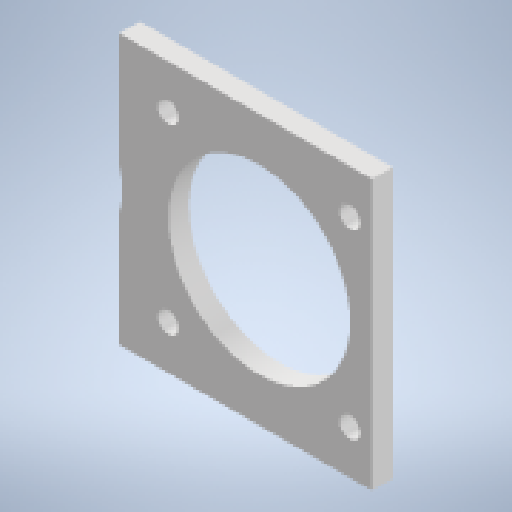
# Autodesk Inventor part: Shaft stabilizer
Saved by Autodesk Inventor 2024 (Build 280153000, 153)
## iProperties
Created: 2024-04-03
Part Number: Shaft stabilizer
Material: Generic
Document SubType Name: Modeling
Designer: drew
Density: 1 g/cm^3
Appearance: Default
Author: drew
Autodesk Inventor part; units mm, degrees
ref_plane "YZ Plane" through (0, 0, 0) normal (1, 0, 0) x (0, 1, 0)
ref_plane "XZ Plane" through (0, 0, 0) normal (0, 1, 0) x (-1, 0, 0)
ref_plane "XY Plane" through (0, 0, 0) normal (0, 0, 1) x (1, 0, 0)
sketch "Sketch1" plane through (0, 0, 0) normal (0, 0, 1) x (1, 0, 0)
  circle A0 centre (17.25, 15.5) radius 1.75 projected
  line L0 (-22.0887, 3.6324) -> (-22.0887, 23) projected
  arc A1 (-22.0887, -3.6324) -> (-22.0887, 3.6324) centre (-33, 0) ccw projected
  line L1 (-22.0887, -23) -> (-22.0887, -3.6324) projected
  line L2 (21, -23) -> (-22.0887, -23) projected
  line L3 (21, 23) -> (21, -23) projected
  line L4 (-22.0887, 23) -> (21, 23) projected
  circle A2 centre (17.25, -15.5) radius 1.75 projected
  circle A3 centre (-13.75, -15.5) radius 1.75 projected
  circle A4 centre (-13.75, 15.5) radius 1.75 projected
  circle A5 centre (17.25, 15.5) radius 1.75 projected
  circle A6 centre (1.75, 0) radius 15.5 projected
  point P0 (0, 0)
extrude "Extrusion1" add sketch "Sketch1" along normal blind 3.5
ref_plane "Work Plane1" through (-33, 0, -23) normal (0, 0, 1) x (1, 0, 0)
sketch "Sketch2" plane through (-33, 0, -23) normal (0, 0, 1) x (1, 0, 0)
  spline S0 degree 3 poles (-10, 18.589) (-10, 18.7259) (-9.9842, 18.8622) (-9.9495, 19.0178) (-9.9443, 19.0395) (-9.8997, 19.2118) (-9.8438, 19.3561) (-9.7735, 19.4974) (-9.7728, 19.4987) (-9.7722, 19.5) knots 0 0 0 0 0.433174 0.433174 0.503481 0.503481 0.995358 0.995358 1 1 1 1
  line L0 (-10, 12.8288) -> (-10, 18.589)
  arc A0 (-15, 7.8288) -> (-10, 12.8288) centre (-15, 12.8288) ccw
  line L1 (-15, 7.8288) -> (-28.448, 7.8288)
  arc A1 (-28.448, 7.8288) -> (-34.7485, 4.6469) centre (-28.448, 0) ccw
  line L2 (-34.7485, 4.6469) -> (-47.9719, -13.2822)
  arc A2 (-47.9719, -13.2822) -> (-48.948, -16.25) centre (-43.948, -16.25) ccw
  line L3 (-48.948, -16.25) -> (-48.948, -47.25)
  arc A3 (-48.948, -47.25) -> (-43.948, -52.25) centre (-43.948, -47.25) ccw
  line L4 (-43.948, -52.25) -> (-13.1315, -52.25)
  arc A4 (-9.9315, -53.4082) -> (-13.1315, -52.25) centre (-13.1315, -57.25) ccw
  arc A5 (8, -43.1993) -> (-9.9315, -53.4082) centre (0, -50) ccw
  line L5 (8, -27) -> (8, -43.1993)
  line L6 (-5.6105, -27) -> (8, -27)
  ellipse E0 centre (-5.6105, -23) end of major axis (-10.9113, -23) minor radius 4 (-10.9113, -23) -> (-5.6105, -27) ccw
  line L7 (-10.9113, -19.5) -> (-10.9113, -23)
  line L8 (8, -19.5) -> (-10.9113, -19.5)
  line L9 (8, -8.2614) -> (8, -19.5)
  arc A6 (8, -8.2614) -> (8, 8.2614) centre (0, 0) ccw
  line L10 (8, 19.5) -> (8, 8.2614)
  line L11 (-9.7722, 19.5) -> (8, 19.5)
  circle A7 centre (0, 8) radius 1.75
  circle A8 centre (0, -8) radius 1.75
  circle A9 centre (0, 0) radius 5.25
  circle A10 centre (-8, 0) radius 1.75
  circle A11 centre (8, 0) radius 1.75
  circle A12 centre (-28.448, -31.75) radius 15.5
  circle A13 centre (-12.948, -16.25) radius 1.75
  circle A14 centre (-43.948, -16.25) radius 1.75
  circle A15 centre (-43.948, -47.25) radius 1.75
  circle A16 centre (-12.948, -47.25) radius 1.75
  circle A17 centre (-28.448, 0) radius 2.55
  line L12 (-13.1315, -51.25) -> (-43.948, -51.25)
  arc A18 (-47.948, -47.25) -> (-43.948, -51.25) centre (-43.948, -47.25) ccw
  line L13 (-47.948, -47.25) -> (-47.948, -16.25)
  arc A19 (-47.1671, -13.8757) -> (-47.948, -16.25) centre (-43.948, -16.25) ccw
  line L14 (-47.1671, -13.8757) -> (-33.9437, 4.0533)
  arc A20 (-28.448, 6.8288) -> (-33.9437, 4.0533) centre (-28.448, 0) ccw
  line L15 (-28.448, 6.8288) -> (-15, 6.8288)
  arc A21 (-15, 6.8288) -> (-9, 12.8288) centre (-15, 12.8288) ccw
  line L16 (-9, 12.8288) -> (-9, 18.5)
  line L17 (-9, 18.5) -> (7, 18.5)
  line L18 (7, 18.5) -> (7, 7.8262)
  arc A22 (7, -7.8262) -> (7, 7.8262) centre (0, 0) ccw
  line L19 (7, -7.8262) -> (7, -18.5)
  line L20 (7, -18.5) -> (-11.9113, -18.5)
  line L21 (-11.9113, -18.5) -> (-11.9113, -23)
  line L22 (-5.6105, -28) -> (7, -28)
  line L23 (7, -28) -> (7, -40.8759)
  arc A23 (7, -40.8759) -> (-11.4011, -51.505) centre (0, -50) ccw
  arc A24 (-11.4011, -51.505) -> (-13.1315, -51.25) centre (-13.1315, -57.25) ccw
  line L24 (-12.948, -16.25) -> (-43.948, -16.25) construction
  line L25 (-12.948, -12.25) -> (-43.948, -12.25)
  arc A25 (-43.948, -12.25) -> (-47.948, -16.25) centre (-43.948, -16.25) ccw
  arc A26 (-8.948, -16.25) -> (-12.948, -12.25) centre (-12.948, -16.25) ccw
  arc A27 (-10.9113, -19.6926) -> (-10.6162, -19.5) centre (-12.948, -16.25) ccw
  line L26 (-8.948, -16.25) -> (-8.948, -18.5)
  line L27 (-8.948, -27.2475) -> (-8.948, -42.7762)
  spline S1 degree 5 poles (-11.9113, -23) (-11.9113, -23.4771) (-11.8403, -23.9542) (-11.6987, -24.4173) (-11.1665, -25.5569) (-10.282, -26.4744) (-9.6463, -26.9319) (-8.4779, -27.5387) (-7.2087, -27.8665) (-6.6793, -27.9555) (-6.1449, -28) (-5.6105, -28) knots 0 0 0 0 0 0 0.267723 0.267723 0.267723 0.700157 0.700157 0.700157 1 1 1 1 1 1
  point P0 (33, 0)
  point P1 (-28.448, -16.25)
  point P2 (-11.2889, -47.8067)
  point P3 (-11.2059, -47.4157)
  point P4 (-47.1671, -13.8757)
  dimension "d2" = 1
  dimension "d3" = 16.948
  constraints: 34 end point, 21 point on circle, 10 centre point, 5 tangent, 3 parallel, 3 point on line, 1 horizontal, 1 midpoint, 1 perpendicular, 1 vertical, 22 other
  measures "d2" distance between parallel lines of L4 L12
  measures "d3" distance between parallel lines of L26 L5
extrude "Extrusion2" add sketch "Sketch2" along normal blind 3.5 contours A16 A23 A24 L12 A18 L13 A19 A25 L25 A26 L26 L20 L21 S1 L27
ref_plane "Work Plane2" through (-33, 0, 34.15) normal (0, 0, 1) x (1, 0, 0)
sketch "Sketch3" plane through (-33, 0, 34.15) normal (0, 0, 1) x (1, 0, 0)
  circle A0 centre (-28.448, 0) radius 2.55 projected
  circle A1 centre (0, 0) radius 5.25 projected
  circle A2 centre (34.75, 0) radius 15.5 projected
  circle A3 centre (-28.448, -31.75) radius 15.5 projected
  circle A4 centre (19.25, -15.5) radius 1.75 projected
  circle A5 centre (19.25, 15.5) radius 1.75 projected
  circle A6 centre (19.25, 15.5) radius 3.175
  circle A7 centre (19.25, -15.5) radius 3.175
  line L0 (54, 23) -> (10.9113, 23) projected
  line L1 (10.9113, -23) -> (54, -23) projected
  line L2 (23.6113, 23) -> (10.9113, 23)
  line L3 (10.9113, 23) -> (10.9113, -23)
  line L4 (10.9113, -23) -> (23.6113, -23)
  line L5 (23.6113, -23) -> (23.6113, 23)
  arc A8 (-30.8569, 5.8754) -> (-34.5684, 1.6919) centre (-28.448, 0) ccw
  line L6 (10.9113, 23) -> (-30.8569, 5.8754)
  arc A9 (-47.948, -47.25) -> (-43.948, -51.25) centre (-43.948, -47.25) ccw projected
  line L7 (-43.948, -51.25) -> (-13.1315, -51.25) projected
  arc A10 (-11.4011, -51.505) -> (-13.1315, -51.25) centre (-13.1315, -57.25) ccw projected
  arc A11 (-11.2889, -47.8067) -> (-11.4011, -51.505) centre (0, -50) ccw projected
  arc A12 (-11.2059, -47.4157) -> (-11.2889, -47.8067) centre (-12.948, -47.25) ccw projected
  arc A13 (-8.948, -42.7762) -> (-11.2059, -47.4157) centre (0, -50) ccw projected
  line L8 (-8.948, -42.7762) -> (-8.948, -27.2475) projected
  line L9 (-11.9113, -23) -> (-11.9113, -18.5) projected
  line L10 (-11.9113, -18.5) -> (-8.948, -18.5) projected
  line L11 (-8.948, -18.5) -> (-8.948, -16.25) projected
  arc A14 (-8.948, -16.25) -> (-12.948, -12.25) centre (-12.948, -16.25) ccw projected
  line L12 (-12.948, -12.25) -> (-43.948, -12.25) projected
  arc A15 (-43.948, -12.25) -> (-47.948, -16.25) centre (-43.948, -16.25) ccw projected
  line L13 (-47.948, -16.25) -> (-47.948, -47.25) projected
  circle A16 centre (-43.948, -47.25) radius 1.75 projected
  circle A17 centre (-43.948, -16.25) radius 1.75 projected
  circle A18 centre (-12.948, -16.25) radius 1.75 projected
  circle A19 centre (-28.448, -31.75) radius 15.5 projected
  circle A20 centre (-43.948, -47.25) radius 3.175
  circle A21 centre (-12.948, -16.25) radius 3.175
  line L14 (-9.2457, -14.7358) -> (-10.5083, -14.2181)
  line L15 (-14.5218, -12.5726) -> (-15.3087, -12.25)
  arc A22 (-47.8034, -46.1842) -> (-42.0904, -50.7925) centre (-43.948, -47.25) ccw
  line L16 (-34.5684, 1.6919) -> (-47.8034, -46.1842)
  line L17 (10.9113, -23) -> (-42.0904, -50.7925)
  point P0 (33, 0)
  point P1 (-10.7079, -18.5)
  point P2 (-47.948, -47.25)
  point P3 (10.9113, 23)
  dimension "d12" = 6.35
  dimension "d6" = 6.35
  dimension "d7" = 6.35
  dimension "d8" = 12.7
  dimension "d9" = 12.7
  dimension "d11" = 6.35
  constraints: 18 end point, 6 coincident, 6 point on circle, 6 tangent, 5 centre point, 2 parallel, 2 point on line, 1 collinear, 1 concentric, 1 horizontal, 1 perpendicular, 4 other
  measures "d6" diameter of A6
  measures "d7" diameter of A7
  measures "d8" diameter of A8
  measures "d9" distance between parallel lines of L5 L3
  measures "d11" diameter of A20
extrude "Extrusion3" add sketch "Sketch3" along normal blind 3.5 contours L5 A2 | A2 L5 L1 L3 L0 | L3 L17 A3 L16 A8 L6 | L17 A3 L16 | L17 A22 A9 L16 A3 picked at (22.1887, -0.5664)
sketch "Sketch4" plane through (-22.0887, 23, 34.15) normal (0, 1, 0) x (1, 0, 0)
  line L0 (12.7, 0) -> (12.7, -3.5) projected
  line L1 (0, 30.65) -> (43.0887, 30.65) projected
  line L2 (12.7, -3.5) -> (43.0887, 30.65)
  line L3 (0, 0) -> (12.7, 17.95)
  line L4 (12.7, 17.95) -> (12.7, 30.65)
  line L5 (12.7, 0) -> (0, 0) projected
  point P0 (22.0887, 34.15)
  dimension "d15" = 12.7
  dimension "d16" = 12.7
  constraints: 6 end point, 1 coincident, 1 perpendicular, 1 point on line
  measures "d15" distance from line of L1.start L4
  measures "d16" distance from line of L1 L3.end
extrude "Extrusion4" add sketch "Sketch4" against normal blind 3.5
mirror "Mirror1" about plane through (0, 0, 0) normal (0, 1, 0) of "Extrusion4"
sketch "Sketch5" plane through (-33, 0, -19.5) normal (0, 0, 1) x (1, 0, 0)
  arc A0 (-47.948, -47.25) -> (-43.948, -51.25) centre (-43.948, -47.25) ccw projected
  line L0 (-43.948, -51.25) -> (-13.1315, -51.25) projected
  arc A1 (-11.4011, -51.505) -> (-13.1315, -51.25) centre (-13.1315, -57.25) ccw projected
  arc A2 (-11.2889, -47.8067) -> (-11.4011, -51.505) centre (0, -50) ccw projected
  arc A3 (-11.2059, -47.4157) -> (-11.2889, -47.8067) centre (-12.948, -47.25) ccw projected
  arc A4 (-8.948, -42.7762) -> (-11.2059, -47.4157) centre (0, -50) ccw projected
  line L1 (-8.948, -42.7762) -> (-8.948, -27.2475) projected
  spline S0 degree 5 poles (-8.948, -27.2475) (-9.4997, -26.9759) (-10.0205, -26.6413) (-10.4974, -26.2419) (-11.2329, -25.4146) (-11.6987, -24.4173) (-11.8403, -23.9542) (-11.9113, -23.4771) (-11.9113, -23) knots 0 0 0 0 0 0 0.563078 0.563078 0.563078 1 1 1 1 1 1 projected
  line L2 (-11.9113, -23) -> (-11.9113, -18.5) projected
  line L3 (-11.9113, -18.5) -> (-8.948, -18.5) projected
  line L4 (-8.948, -18.5) -> (-8.948, -16.25) projected
  arc A5 (-8.948, -16.25) -> (-12.948, -12.25) centre (-12.948, -16.25) ccw projected
  line L5 (-12.948, -12.25) -> (-43.948, -12.25) projected
  arc A6 (-43.948, -12.25) -> (-47.948, -16.25) centre (-43.948, -16.25) ccw projected
  line L6 (-47.948, -16.25) -> (-47.948, -47.25) projected
  circle A7 centre (-43.948, -47.25) radius 1.75 projected
  circle A8 centre (-43.948, -16.25) radius 1.75 projected
  circle A9 centre (-12.948, -16.25) radius 1.75 projected
  circle A10 centre (-28.448, -31.75) radius 15.5 projected
  arc A11 (-47.8034, -46.1842) -> (-42.0904, -50.7925) centre (-43.948, -47.25) ccw projected
  line L7 (-42.0904, -50.7925) -> (10.9113, -23) projected
  line L8 (10.9113, -23) -> (23.6113, -23) projected
  line L9 (23.6113, -23) -> (23.6113, -19.5) projected
  line L10 (23.6113, -19.5) -> (23.6113, 19.5) projected
  line L11 (23.6113, 19.5) -> (23.6113, 23) projected
  line L12 (23.6113, 23) -> (10.9113, 23) projected
  line L13 (10.9113, 23) -> (-30.8569, 5.8754) projected
  arc A12 (-30.8569, 5.8754) -> (-34.5684, 1.6919) centre (-28.448, 0) ccw projected
  line L14 (-34.5684, 1.6919) -> (-47.8034, -46.1842) projected
  circle A13 centre (-43.948, -47.25) radius 3.175 projected
  arc A14 (-8.948, -16.25) -> (-9.2457, -14.7358) centre (-12.948, -16.25) ccw projected
  line L15 (-8.948, -16.25) -> (-8.948, -18.5) projected
  line L16 (-8.948, -18.5) -> (-10.7079, -18.5) projected
  arc A15 (-10.5083, -14.2181) -> (-10.7079, -18.5) centre (-12.948, -16.25) ccw projected
  line L17 (-10.5083, -14.2181) -> (-9.2457, -14.7358) projected
  circle A16 centre (-28.448, 0) radius 2.55 projected
  circle A17 centre (0, 0) radius 5.25 projected
  circle A18 centre (19.25, -15.5) radius 3.175 projected
  circle A19 centre (19.25, 15.5) radius 3.175 projected
  circle A20 centre (-28.448, 0) radius 25.4
  circle A21 centre (-28.448, -31.75) radius 6.35
  circle A22 centre (-28.448, 0) radius 29.4
  point P0 (33, 0)
  point P1 (-43.9411, -32.2127)
  point P2 (-47.948, -47.25)
  point P3 (-33.6323, -46.3573)
  point P4 (-11.7335, -24.1864)
  point P5 (-14.176, -25.7035)
  point P6 (-13.4844, -35.7924)
  point P7 (-8.948, -33.4136)
  dimension "d19" = 50.8
  dimension "d20" = 12.7
  dimension "d21" = 4
  constraints: 3 centre point, 2 coincident, 1 other
  measures "d19" diameter of A20
  measures "d20" diameter of A21
  measures "d21" radial gap between concentric circles of A20 A22
extrude "Extrusion5" add sketch "Sketch5" along normal up to surface (53.65 mm away) contours A11 L14 A10 L7 A0 | A10 A22 S0 L1 L7
body "Solid1"
